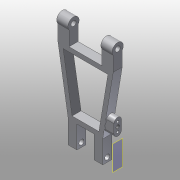
# Autodesk Inventor part: 500-006
Saved by Autodesk Inventor 2016 (Build 200138000, 138)
## iProperties
Created: 2015-04-18
Part Number: 500-006
Material: ABS Plastic
Document SubType Name: Modeling
Designer: Station9
Density: 1.06 g/cm^3
Appearance: Smooth - White
Mass: 5.1553 g
Surface Area: 43.8752 cm^2
Volume: 4.86349 cm^3
Author: Station9
Autodesk Inventor part; units mm, degrees
ref_plane "YZ Plane" through (0, 0, 0) normal (1, 0, 0) x (0, 1, 0)
ref_plane "XZ Plane" through (0, 0, 0) normal (0, 1, 0) x (-1, 0, 0)
ref_plane "XY Plane" through (0, 0, 0) normal (0, 0, 1) x (1, 0, 0)
sketch "Sketch1" plane through (0, 0, 0) normal (0, 1, 0) x (-1, 0, 0)
  line L0 (11, 32.7929) -> (11, 17.7929)
  line L1 (11, 17.7929) -> (-2.062, 17.7929)
  line L2 (11, 32.7929) -> (18.5, 32.7929)
  line L3 (18.5, 32.7929) -> (18.5, 17.7929)
  line L4 (18.5, 17.7929) -> (11.5, -24.2071)
  line L5 (11.5, -24.2071) -> (11.5, -39.2071)
  line L6 (11.5, -39.2071) -> (5.7, -39.2071)
  line L7 (5.7, -39.2071) -> (5.7, -24.2071)
  line L8 (5.7, -24.2071) -> (0.6352, -24.2071)
  line L9 (0, 0) -> (0, 4.5611)
  line L10 (-11, 32.7929) -> (-11, 17.7929)
  line L11 (-11, 17.7929) -> (-2.062, 17.7929)
  line L12 (-11, 32.7929) -> (-18.5, 32.7929)
  line L13 (-18.5, 32.7929) -> (-18.5, 17.7929)
  line L14 (-18.5, 17.7929) -> (-11.5, -24.2071)
  line L15 (-11.5, -24.2071) -> (-11.5, -39.2071)
  line L16 (-11.5, -39.2071) -> (-5.7, -39.2071)
  line L17 (-5.7, -39.2071) -> (-5.7, -24.2071)
  line L18 (-5.7, -24.2071) -> (0.6352, -24.2071)
  dimension "d0" = 37
  dimension "d1" = 7.5
  dimension "d2" = 15
  dimension "d3" = 5.8
  dimension "d4" = 23
  dimension "d5" = 72
  dimension "d6" = 15
  dimension "d7" = 15
  dimension "d8" = 15
  constraints: 38 end point, 8 symmetric about line, 5 perpendicular, 2 vertical, 1 horizontal, 1 parallel
  measures "d0" distance between parallel lines of L13 L3
  measures "d1" distance between parallel lines of L3 L0
  measures "d2" distance of L0.start L0.end
  measures "d3" distance of L5.end L6.end
  measures "d4" distance between parallel lines of L15 L5
  measures "d5" distance between parallel lines of L2 L6
  measures "d6" distance of L6.end L7.end
  measures "d7" distance of L2.end L3.end
  measures "d8" distance of L4.end L5.end
extrude "Extrusion1" add sketch "Sketch1" along normal blind 6
sketch "Sketch2" plane through (0, 6, 0) normal (0, 1, 0) x (1, 0, 0)
  line L0 (-11, -17.7929) -> (11, -17.7929) projected
  line L1 (18.5, -17.7929) -> (11.5, 24.2071) projected
  line L2 (5.7, 24.2071) -> (-5.7, 24.2071) projected
  line L3 (-11.5, 24.2071) -> (-18.5, -17.7929) projected
  line L4 (-14.9586, -14.7929) -> (-8.9586, 21.2071)
  line L5 (-8.9586, 21.2071) -> (8.9586, 21.2071)
  line L6 (8.9586, 21.2071) -> (14.9586, -14.7929)
  line L7 (14.9586, -14.7929) -> (-14.9586, -14.7929)
  point P0 (0, 0)
  dimension "d11" = 3
  dimension "d12" = 3
  dimension "d13" = 3
  dimension "d14" = 3
  constraints: 8 end point, 1 horizontal, 1 parallel
  measures "d11" distance between parallel lines of L0 L7
  measures "d12" distance between parallel lines of L3 L4
  measures "d13" distance between parallel lines of L6 L1
  measures "d14" distance between parallel lines of L5 L2
extrude "Extrusion2" cut sketch "Sketch2" against normal blind 6
sketch "Sketch3" plane through (-5.7, 0, -24.2071) normal (1, 0, 0) x (0, 0, -1)
  line L0 (15, 0) -> (15, 6) projected
  circle A0 centre (12, 3) radius 1.7
  point P0 (-24.2071, 0)
  dimension "d17" = 3.4
  dimension "d18" = 3
  constraints: 1 centre point
  measures "d17" diameter of A0
  measures "d18" distance from line of L0 A0.centre
extrude "Extrusion3" cut sketch "Sketch3" along normal through all both and the other way through all
sketch "Sketch4" plane through (18.5, 0, 32.7929) normal (1, 0, 0) x (0, 0, -1)
  line L0 (0, 0) -> (0, 6) projected
  circle A0 centre (3, 3) radius 3.75
  point P0 (32.7929, 0)
  dimension "d21" = 7.5
  dimension "d22" = 3
  constraints: 1 centre point
  measures "d21" diameter of A0
  measures "d22" distance from line of A0.centre L0
extrude "Extrusion4" add sketch "Sketch4" against normal up to surface (7.5 mm away)
sketch "Sketch5" plane through (18.5, 0, 17.7929) normal (1, 0, 0) x (0, 0, -1)
  line L0 (-15, 6) -> (-14.25, 6) projected
  line L1 (-15, 0) -> (-15, 0.75) projected
  line L2 (-15, 0) -> (-14.25, 0) projected
  line L3 (-15, 5.25) -> (-15, 6)
  line L4 (-15, 6) -> (-14.25, 6)
  line L5 (-15, 0.75) -> (-15, 0)
  line L6 (-15, 0) -> (-14.25, 0)
  arc A0 (-14.25, 6) -> (-15, 5.25) centre (-12, 3) ccw
  arc A1 (-15, 0.75) -> (-14.25, 0) centre (-12, 3) ccw
  point P0 (17.7929, 0)
  constraints: 10 end point, 5 point on circle, 2 centre point, 2 vertical, 1 coincident, 1 perpendicular
extrude "Extrusion5" cut sketch "Sketch5" against normal through all
sketch "Sketch6" plane through (-11, 0, 17.7929) normal (1, 0, 0) x (0, 0, -1)
  arc A0 (-15, 0.75) -> (-14.25, 0) centre (-12, 3) ccw projected
  circle A1 centre (-12, 3) radius 3.75
  point P0 (17.7929, 0)
  dimension "d27" = 7.5
  constraints: 1 centre point, 1 coincident
  measures "d27" diameter of A1
extrude "Extrusion6" add sketch "Sketch6" against normal up to surface (7.5 mm away)
hole "Hole1" at (18.5, 3, 29.7929) direction (-1, 0, 0) diameter 3.4 depth 46.75 tip angle 118
ref_plane "Work Plane1" through (18.5, 0, -39.2071) normal (-1, 0, 0) x (0, 0, 1)
sketch "Sketch7" plane through (18.5, 0, -39.2071) normal (-1, 0, 0) x (0, 0, 1)
  line L0 (27, 3) -> (21, 3) construction
  line L1 (27, 0.5) -> (21, 0.5)
  line L2 (21, 5.5) -> (27, 5.5)
  arc A0 (27, 0.5) -> (27, 5.5) centre (27, 3) ccw
  arc A1 (21, 5.5) -> (21, 0.5) centre (21, 3) ccw
  circle A2 centre (3, 3) radius 1.7 projected
  line L3 (15, 0) -> (15, 6) projected
  point P0 (39.2071, 0)
  point P1 (24, 3)
  point P2 (15, 3)
  dimension "d40" = 21
  dimension "d41" = 5
  dimension "d42" = 6
  constraints: 8 end point, 4 point on circle, 4 tangent, 2 centre point, 2 midpoint, 1 horizontal, 1 horizontal alignment, 1 parallel
  measures "d40" distance of point (24, 3) A2.centre
  measures "d41" distance between parallel lines of L1 L2
  measures "d42" distance of L0.start L0.end
extrude "Extrusion7" add sketch "Sketch7" along normal blind 7.25 contours L1 A1 L2 A0
sketch "Sketch8" plane through (18.5, 0, -39.2071) normal (1, 0, 0) x (0, 0, -1)
  arc A0 (-21, 0.5) -> (-21, 5.5) centre (-21, 3) ccw projected
  arc A1 (-27, 5.5) -> (-27, 0.5) centre (-27, 3) ccw projected
  point P0 (-39.2071, 0)
hole "Hole2" at (18.5, 3, -12.2071) at (18.5, 3, -18.2071) direction (-1, 0, 0) diameter 1.5 depth 3 tip angle 118
sketch "Sketch9" plane through (18.5, 0, -39.2071) normal (1, 0, 0) x (0, 0, -1)
  arc A0 (-21, 0.5) -> (-21, 5.5) centre (-21, 3) ccw projected
  arc A1 (-27, 5.5) -> (-27, 0.5) centre (-27, 3) ccw projected
  line L0 (-27, 3) -> (-21, 3)
  point P0 (-39.2071, 0)
  point P1 (-24, 3)
  constraints: 2 end point, 1 horizontal, 1 midpoint
hole "Hole3" at (18.5, 3, -15.2071) direction (-1, 0, 0) diameter 2.459 depth 10.8 tip angle 118 thread size "M3x0.5" class "6H" standard "ISO Metric profile"
equation "\"d8\" = d7"
body "Solid1"
